Autodesk Inventor part; units mm, degrees
(part 3 of 3)
  line L283 (26.9505, 35.0379) -> (29.2108, 35.0457)
  line L284 (31.5582, 39.3166) -> (31.5476, 42.4293)
  line L285 (31.5596, 38.9092) -> (26.3728, 35.924)
  line L286 (26.3714, 36.3314) -> (31.5582, 39.3166)
  line L287 (31.5476, 42.4293) -> (21.5221, 36.4783)
  line L288 (31.7603, 43.0725) -> (21.0767, 36.7309)
  line L289 (19.9586, 37.4674) -> (31.7966, 44.45)
  line L290 (31.9286, 42.4307) -> (31.9366, 40.0825)
  line L291 (31.9286, 42.4307) -> (31.9285, 42.4639)
  line L292 (31.7966, 44.45) -> (43.6866, 37.5937)
  line L293 (42.5183, 36.9086) -> (31.7603, 43.0725)
  line L294 (42.0747, 36.6505) -> (31.9285, 42.4639)
  line L295 (31.5636, 37.7372) -> (31.5596, 38.9092)
  arc A47 (31.5636, 37.7372) -> (31.9446, 37.7385) centre (31.7568, 36.9673) ccw
  line L296 (38.1142, 35.719) -> (38.1116, 36.4859)
  arc A48 (38.7601, 35.0783) -> (38.1142, 35.719) centre (37.9285, 34.8858) ccw
  line L297 (37.7332, 36.2932) -> (37.7351, 35.7209)
  line L298 (38.3728, 25.9055) -> (37.1595, 25.9014)
  line L299 (37.1582, 26.2824) -> (38.3715, 26.2865)
  line L300 (37.1595, 25.9014) -> (37.1582, 26.2824)
  line L301 (36.3108, 29.8585) -> (35.1678, 29.8546)
  line L302 (34.347, 26.7047) -> (35.1786, 26.7075)
  line L303 (35.1678, 29.8546) -> (35.1786, 26.7075)
  line L304 (35.1786, 26.7075) -> (35.2746, 26.7079)
  line L305 (36.3215, 26.7115) -> (36.3108, 29.8585)
  line L306 (36.3215, 26.7115) -> (37.1567, 26.7143)
  line L307 (34.3505, 25.6887) -> (34.347, 26.7047)
  line L308 (37.1602, 25.6983) -> (34.3505, 25.6887)
  line L309 (37.1567, 26.7143) -> (37.1602, 25.6983)
  arc A49 (38.6709, 29.0181) -> (38.3681, 27.268) centre (38.5556, 28.1368) ccw
  line L310 (29.165, 23.8796) -> (25.8795, 23.8684)
  line L311 (23.0676, 23.4777) -> (29.1663, 23.4986)
  line L312 (30.8931, 30.8743) -> (32.1631, 30.8786)
  line L313 (33.9093, 28.7073) -> (32.6624, 28.703)
  line L314 (32.6638, 28.2849) -> (32.6624, 28.703)
  line L315 (33.9107, 28.2892) -> (32.6638, 28.2849)
  line L316 (33.9142, 27.2732) -> (33.9107, 28.2892)
  line L317 (32.6585, 29.846) -> (31.5155, 29.8421)
  line L318 (31.5155, 29.8421) -> (33.9054, 29.8503)
  line L319 (31.5194, 28.6991) -> (31.5155, 29.8421)
  line L320 (32.6673, 27.2689) -> (33.9142, 27.2732)
  line L321 (32.6688, 26.818) -> (32.6673, 27.2689)
  line L322 (33.9158, 26.8222) -> (32.6688, 26.818)
  line L323 (31.5155, 29.8421) -> (31.5298, 25.6711)
  line L324 (33.9197, 25.6792) -> (33.9158, 26.8222)
  line L325 (31.5298, 25.6711) -> (33.9197, 25.6792)
  line L326 (31.5298, 25.6711) -> (32.6728, 25.675)
  line L327 (31.5258, 26.8141) -> (31.5298, 25.6711)
  line L328 (31.5208, 28.281) -> (31.5243, 27.265)
  line L329 (39.2326, 22.7164) -> (42.1166, 24.4043)
  line L330 (38.7647, 22.7148) -> (39.2326, 22.7164)
  line L331 (35.6693, 22.7042) -> (38.3837, 22.7135)
  line L332 (35.2848, 23.7486) -> (35.2883, 22.7029)
  circle A50 centre (35.4727, 24.4871) radius 0.3175
  arc A51 (35.6658, 23.7499) -> (35.2848, 23.7486) centre (35.4727, 24.4871) ccw
  line L333 (32.0618, 22.6919) -> (35.2883, 22.7029)
  line L334 (35.6693, 22.7042) -> (35.6658, 23.7499)
  line L335 (38.5779, 22.3332) -> (32.0667, 22.3109)
  line L336 (32.0667, 22.3109) -> (38.5779, 22.3332)
  line L337 (31.8964, 17.907) -> (42.562, 24.1393)
  line L338 (43.6957, 23.5059) -> (31.8713, 16.6404)
  line L339 (32.0796, 18.5298) -> (38.5779, 22.3332)
  line L340 (32.0761, 18.5277) -> (38.5779, 22.3332)
  line L341 (32.0667, 22.3109) -> (32.0796, 18.5298)
  line L342 (31.75, 80.4139) -> (44.6823, 72.8573)
  line L343 (44.6823, 72.8573) -> (54.0323, 76.3351)
  line L344 (54.0323, 76.3351) -> (63.5, 70.8029)
  line L345 (31.75, 72.2052) -> (31.75, 88.9) construction
  line L346 (31.75, 80.4139) -> (18.8177, 72.8573)
  line L347 (18.8177, 72.8573) -> (9.4677, 76.3351)
  line L348 (9.4677, 76.3351) -> (0, 70.8029)
  line L349 (29.1432, 44.45) -> (63.5, 44.45) construction
  line L350 (9.4677, 12.5649) -> (0, 18.0971)
  line L351 (18.8177, 16.0427) -> (9.4677, 12.5649)
  line L352 (31.75, 8.4861) -> (18.8177, 16.0427)
  line L353 (31.75, 8.4861) -> (44.6823, 16.0427)
  line L354 (44.6823, 16.0427) -> (54.0323, 12.5649)
  line L355 (54.0323, 12.5649) -> (63.5, 18.0971)
  line L356 (0, 51.1737) -> (17.8526, 51.1737)
  line L357 (17.8526, 51.1737) -> (29.1432, 44.45)
  line L358 (17.8526, 37.7263) -> (29.1432, 44.45)
  line L359 (0, 37.7263) -> (17.8526, 37.7263)
  line L360 (63.5, 51.1737) -> (45.6474, 51.1737)
  line L361 (45.6474, 51.1737) -> (34.3568, 44.45)
  line L362 (45.6474, 37.7263) -> (34.3568, 44.45)
  line L363 (63.5, 37.7263) -> (45.6474, 37.7263)
  point P0 (0, 0)
  point P1 (31.7785, 58.3278)
  point P2 (31.8262, 30.4638)
  point P3 (-150.7587, 38.3711)
  point P4 (-161.1855, 44.542)
  point P5 (-156.3366, 47.458)
  point P6 (-155.762, 47.458)
  point P7 (-155.762, 49.0926)
  point P8 (-150.6894, 62.2724)
  point P9 (-155.762, 49.4736)
  point P10 (-154.619, 45.7468)
  point P11 (-155.762, 46.7628)
  point P12 (-155.762, 47.077)
  point P13 (-145.5843, 54.5372)
  point P14 (-145.5843, 54.9182)
  point P15 (-155.762, 53.9477)
  point P16 (-155.762, 53.5667)
  point P17 (-150.0718, 50.9582)
  point P18 (-151.2148, 52.1012)
  point P19 (-151.2148, 52.5193)
  point P20 (-150.7519, 34.4405)
  point P21 (-161.1576, 28.2339)
  point P22 (-155.7186, 23.702)
  point P23 (-155.7242, 25.3366)
  point P24 (-156.2988, 25.3346)
  point P25 (-155.7033, 19.2279)
  point P26 (-155.702, 18.8469)
  point P27 (-145.521, 17.9112)
  point P28 (-145.5223, 18.2922)
  point P29 (-155.7255, 25.7176)
  point P30 (-155.7266, 26.0318)
  point P31 (-154.587, 27.0517)
  point P32 (-155.7173, 23.321)
  point P33 (-151.1611, 20.7089)
  point P34 (-150.022, 21.8558)
  point P35 (-119.1805, 10.1069)
  point P36 (-182.6805, 10.1069)
  point P37 (-182.6805, 62.8127)
  dimension "d27" = 63.5
  dimension "d28" = 88.9
  constraints: 728 end point, 89 parallel, 64 point on circle, 50 centre point, 37 horizontal, 22 point on line, 21 perpendicular, 20 coincident, 17 symmetric about line, 5 vertical, 4 collinear, 2 midpoint, 11 other
  measures "d27" distance of L2.end L1.end
  measures "d28" distance of L1.end L0.end
extrude "Extrusion5" add sketch "Sketch6" against normal blind 0.8 separate body contours L109 L133 L129 L127 L155 L144 | L288 L293 L207 L337 L189 L182
sketch "Sketch7" plane through (0, 0, 0.4) normal (0, 0, 1) x (1, 0, 0)
  line L0 (63.5, 0) -> (63.5, 18.0971) projected
  line L1 (63.5, 0) -> (0, 0)
  line L2 (0, 0) -> (0, 88.9)
  line L3 (0, 88.9) -> (63.5, 88.9)
  line L4 (63.5, 88.9) -> (63.5, 0)
  constraints: 8 end point, 2 parallel, 1 horizontal, 1 perpendicular
extrude "Extrusion6" add sketch "Sketch7" along normal blind 0.4 bodies 2
sketch "Sketch8" plane through (0, 0, 0.8) normal (0, 0, 1) x (1, 0, 0)
  line L0 (5.5444, 85.725) -> (13.9597, 85.725) construction
  line L1 (13.9597, 85.725) -> (13.9597, 77.1126) construction
  line L2 (13.9597, 77.1126) -> (5.5444, 77.1126) construction
  line L3 (5.5444, 77.1126) -> (5.5444, 85.725) construction
  line L4 (49.5403, 22.4335) -> (53.7479, 24.8628)
  line L5 (53.7479, 24.8628) -> (57.9556, 22.4335)
  line L6 (57.9556, 22.4335) -> (57.9556, 17.5749)
  line L7 (57.9556, 17.5749) -> (53.7479, 15.1456)
  line L8 (53.7479, 15.1456) -> (49.5403, 17.5749)
  line L9 (49.5403, 17.5749) -> (49.5403, 22.4335)
  line L10 (63.5, 88.9) -> (0, 88.9) construction
  line L11 (63.5, 51.1737) -> (63.5, 37.7263) construction
  line L12 (63.5, 44.45) -> (0, 44.45) construction
  line L13 (0, 37.7263) -> (0, 51.1737) construction
  line L14 (0, 0) -> (63.5, 0) construction
  line L15 (31.75, 0) -> (31.75, 88.9) construction
  line L16 (13.9597, 71.3251) -> (13.9597, 66.4665)
  line L17 (5.5444, 66.4665) -> (5.5444, 71.3251)
  line L18 (13.9597, 66.4665) -> (9.7521, 64.0372)
  line L19 (9.7521, 64.0372) -> (5.5444, 66.4665)
  line L20 (5.5444, 71.3251) -> (9.7521, 73.7544)
  line L21 (9.7521, 73.7544) -> (13.9597, 71.3251)
  line L22 (57.9556, 3.175) -> (49.5403, 3.175) construction
  line L23 (49.5403, 3.175) -> (49.5403, 13.0967) construction
  line L24 (49.5403, 13.0967) -> (57.9556, 13.0967) construction
  line L25 (57.9556, 13.0967) -> (57.9556, 3.175) construction
  line L26 (23.2632, 24.9041) -> (31.75, 29.804)
  line L27 (31.75, 29.804) -> (40.2368, 24.9041)
  line L28 (40.2368, 24.9041) -> (40.2368, 15.1043)
  line L29 (40.2368, 15.1043) -> (31.75, 10.2044)
  line L30 (31.75, 10.2044) -> (23.2632, 15.1043)
  line L31 (23.2632, 15.1043) -> (23.2632, 24.9041)
  line L32 (40.2368, 73.7957) -> (31.75, 78.6956)
  line L33 (31.75, 78.6956) -> (23.2632, 73.7957)
  line L34 (23.2632, 63.9959) -> (31.75, 59.096)
  line L35 (23.2632, 73.7957) -> (23.2632, 63.9959)
  line L36 (31.75, 59.096) -> (40.2368, 63.9959)
  line L37 (40.2368, 63.9959) -> (40.2368, 73.7957)
  line L38 (12.9466, 76.2318) -> (6.681, 76.2318)
  line L39 (6.681, 76.2318) -> (6.681, 77.6726)
  spline S0 degree 2 poles (6.681, 77.6726) (7.3561, 78.3066) (8.5582, 79.484) (9.1346, 80.1179) knots 0 0 0 1 2 2 2
  spline S1 degree 2 poles (9.1346, 80.1179) (10.2955, 81.3941) (11.1435, 82.9255) (11.1435, 83.7406) knots 0 0 0 1 2 2 2
  spline S2 degree 2 poles (11.1435, 83.7406) (11.1435, 84.1688) (10.88, 84.811) (10.6413, 85.0168) knots 0 0 0 1 2 2 2
  spline S3 degree 2 poles (10.6413, 85.0168) (10.4025, 85.2226) (9.7768, 85.4285) (9.398, 85.4285) knots 0 0 0 1 2 2 2
  spline S4 degree 2 poles (9.398, 85.4285) (9.0358, 85.4285) (8.2948, 85.2473) (7.9572, 85.1074) knots 0 0 0 1 2 2 2
  spline S5 degree 2 poles (7.9572, 85.1074) (7.669, 84.9921) (7.1338, 84.6628) (6.9692, 84.5475) knots 0 0 0 1 2 2 2
  line L40 (6.9692, 84.5475) -> (6.8951, 84.5475)
  line L41 (6.8951, 84.5475) -> (6.8951, 85.9966)
  spline S6 degree 2 poles (6.8951, 85.9966) (7.315, 86.2024) (8.8217, 86.6059) (9.4968, 86.6059) knots 0 0 0 1 2 2 2
  spline S7 degree 2 poles (9.4968, 86.6059) (10.9212, 86.6059) (12.5267, 85.0991) (12.5267, 83.8147) knots 0 0 0 1 2 2 2
  spline S8 degree 2 poles (12.5267, 83.8147) (12.5267, 83.2137) (12.2468, 82.2092) (11.9998, 81.7811) knots 0 0 0 1 2 2 2
  spline S9 degree 2 poles (11.9998, 81.7811) (11.7528, 81.3365) (11.0365, 80.4637) (10.6413, 80.0438) knots 0 0 0 1 2 2 2
  spline S10 degree 2 poles (10.6413, 80.0438) (9.9991, 79.344) (8.4265, 77.8455) (7.9572, 77.4092) knots 0 0 0 1 2 2 2
  line L42 (7.9572, 77.4092) -> (12.9466, 77.4092)
  line L43 (12.9466, 77.4092) -> (12.9466, 76.2318)
  line L44 (50.5534, 13.3229) -> (56.819, 13.3229)
  line L45 (56.819, 13.3229) -> (56.819, 11.882)
  spline S11 degree 2 poles (56.819, 11.882) (56.1439, 11.2481) (54.9418, 10.0707) (54.3654, 9.4367) knots 0 0 0 1 2 2 2
  spline S12 degree 2 poles (54.3654, 9.4367) (53.2045, 8.1605) (52.3565, 6.6291) (52.3565, 5.814) knots 0 0 0 1 2 2 2
  spline S13 degree 2 poles (52.3565, 5.814) (52.3565, 5.3859) (52.62, 4.7437) (52.8587, 4.5378) knots 0 0 0 1 2 2 2
  spline S14 degree 2 poles (52.8587, 4.5378) (53.0975, 4.332) (53.7232, 4.1262) (54.102, 4.1262) knots 0 0 0 1 2 2 2
  spline S15 degree 2 poles (54.102, 4.1262) (54.4642, 4.1262) (55.2052, 4.3073) (55.5428, 4.4473) knots 0 0 0 1 2 2 2
  spline S16 degree 2 poles (55.5428, 4.4473) (55.831, 4.5625) (56.3662, 4.8919) (56.5308, 5.0072) knots 0 0 0 1 2 2 2
  line L46 (56.5308, 5.0072) -> (56.6049, 5.0072)
  line L47 (56.6049, 5.0072) -> (56.6049, 3.5581)
  spline S17 degree 2 poles (56.6049, 3.5581) (56.185, 3.3522) (54.6783, 2.9488) (54.0032, 2.9488) knots 0 0 0 1 2 2 2
  spline S18 degree 2 poles (54.0032, 2.9488) (52.5788, 2.9488) (50.9733, 4.4555) (50.9733, 5.7399) knots 0 0 0 1 2 2 2
  spline S19 degree 2 poles (50.9733, 5.7399) (50.9733, 6.341) (51.2532, 7.3454) (51.5002, 7.7736) knots 0 0 0 1 2 2 2
  spline S20 degree 2 poles (51.5002, 7.7736) (51.7472, 8.2182) (52.4635, 9.0909) (52.8587, 9.5108) knots 0 0 0 1 2 2 2
  spline S21 degree 2 poles (52.8587, 9.5108) (53.5009, 10.2107) (55.0735, 11.7091) (55.5428, 12.1455) knots 0 0 0 1 2 2 2
  line L48 (55.5428, 12.1455) -> (50.5534, 12.1455)
  line L49 (50.5534, 12.1455) -> (50.5534, 13.3229)
  point P0 (53.7479, 20.0042)
  point P1 (9.7521, 68.8958)
  point P2 (49.5403, 8.1358)
  point P3 (31.75, 20.0042)
  point P4 (31.75, 68.8958)
  dimension "d33" = 8.4153
  dimension "d34" = 8.4153
  dimension "d35" = 8.4153
  dimension "d41" = 3.175
  dimension "d42" = 3.175
  constraints: 52 end point, 7 symmetric about line, 5 midpoint, 4 vertical, 3 collinear, 1 point on line, 30 other
  measures "d33" distance between parallel lines of L3 L1
  measures "d34" distance between parallel lines of L17 L16
  measures "d35" distance from line of point (49.54, 8.136) L25
  measures "d41" distance between parallel lines of L10 L0
  measures "d42" distance between parallel lines of L14 L22
extrude "Extrusion7" cut sketch "Sketch8" against normal blind 0.4 bodies 2
sketch "Sketch9" plane through (0, 0, 0.4) normal (0, 0, 1) x (1, 0, 0)
  line L0 (12.9466, 77.4092) -> (12.9466, 76.2318) projected
  line L1 (12.9466, 76.2318) -> (6.681, 76.2318) projected
  line L2 (6.681, 76.2318) -> (6.681, 77.6726) projected
  spline S0 degree 2 poles (6.681, 77.6726) (7.3561, 78.3066) (8.5582, 79.484) (9.1346, 80.1179) knots 0 0 0 0.5 1 1 1 projected
  spline S1 degree 2 poles (9.1346, 80.1179) (10.2955, 81.3941) (11.1435, 82.9255) (11.1435, 83.7406) knots 0 0 0 0.5 1 1 1 projected
  spline S2 degree 2 poles (11.1435, 83.7406) (11.1435, 84.1688) (10.88, 84.811) (10.6413, 85.0168) knots 0 0 0 0.5 1 1 1 projected
  spline S3 degree 2 poles (10.6413, 85.0168) (10.4025, 85.2226) (9.7768, 85.4285) (9.398, 85.4285) knots 0 0 0 0.5 1 1 1 projected
  spline S4 degree 2 poles (9.398, 85.4285) (9.0358, 85.4285) (8.2948, 85.2473) (7.9572, 85.1074) knots 0 0 0 0.5 1 1 1 projected
  spline S5 degree 2 poles (7.9572, 85.1074) (7.669, 84.9921) (7.1338, 84.6628) (6.9692, 84.5475) knots 0 0 0 0.5 1 1 1 projected
  line L3 (6.9692, 84.5475) -> (6.8951, 84.5475) projected
  line L4 (6.8951, 84.5475) -> (6.8951, 85.9966) projected
  spline S6 degree 2 poles (6.8951, 85.9966) (7.315, 86.2024) (8.8217, 86.6059) (9.4968, 86.6059) knots 0 0 0 0.5 1 1 1 projected
  spline S7 degree 2 poles (9.4968, 86.6059) (10.9212, 86.6059) (12.5267, 85.0991) (12.5267, 83.8147) knots 0 0 0 0.5 1 1 1 projected
  spline S8 degree 2 poles (12.5267, 83.8147) (12.5267, 83.2137) (12.2468, 82.2092) (11.9998, 81.7811) knots 0 0 0 0.5 1 1 1 projected
  spline S9 degree 2 poles (11.9998, 81.7811) (11.7528, 81.3365) (11.0365, 80.4637) (10.6413, 80.0438) knots 0 0 0 0.5 1 1 1 projected
  spline S10 degree 2 poles (10.6413, 80.0438) (9.9991, 79.344) (8.4265, 77.8455) (7.9572, 77.4092) knots 0 0 0 0.5 1 1 1 projected
  line L5 (7.9572, 77.4092) -> (12.9466, 77.4092) projected
  line L6 (23.2632, 24.9041) -> (31.75, 29.804) projected
  line L7 (31.75, 29.804) -> (40.2368, 24.9041) projected
  line L8 (40.2368, 24.9041) -> (40.2368, 15.1043) projected
  line L9 (40.2368, 15.1043) -> (31.75, 10.2044) projected
  line L10 (31.75, 10.2044) -> (23.2632, 15.1043) projected
  line L11 (23.2632, 15.1043) -> (23.2632, 24.9041) projected
  line L12 (9.7521, 73.7544) -> (13.9597, 71.3251) projected
  line L13 (13.9597, 71.3251) -> (13.9597, 66.4665) projected
  line L14 (13.9597, 66.4665) -> (9.7521, 64.0372) projected
  line L15 (9.7521, 64.0372) -> (5.5444, 66.4665) projected
  line L16 (5.5444, 66.4665) -> (5.5444, 71.3251) projected
  line L17 (5.5444, 71.3251) -> (9.7521, 73.7544) projected
  line L18 (57.9556, 17.5749) -> (53.7479, 15.1456) projected
  line L19 (53.7479, 15.1456) -> (49.5403, 17.5749) projected
  line L20 (49.5403, 17.5749) -> (49.5403, 22.4335) projected
  line L21 (49.5403, 22.4335) -> (53.7479, 24.8628) projected
  line L22 (53.7479, 24.8628) -> (57.9556, 22.4335) projected
  line L23 (57.9556, 22.4335) -> (57.9556, 17.5749) projected
  line L24 (31.75, 78.6956) -> (40.2368, 73.7957) projected
  line L25 (40.2368, 73.7957) -> (40.2368, 63.9959) projected
  line L26 (40.2368, 63.9959) -> (31.75, 59.096) projected
  line L27 (31.75, 59.096) -> (23.2632, 63.9959) projected
  line L28 (23.2632, 63.9959) -> (23.2632, 73.7957) projected
  line L29 (23.2632, 73.7957) -> (31.75, 78.6956) projected
  line L30 (50.5534, 12.1455) -> (50.5534, 13.3229) projected
  line L31 (50.5534, 13.3229) -> (56.819, 13.3229) projected
  line L32 (56.819, 13.3229) -> (56.819, 11.882) projected
  spline S11 degree 2 poles (56.819, 11.882) (56.1439, 11.2481) (54.9418, 10.0707) (54.3654, 9.4367) knots 0 0 0 0.5 1 1 1 projected
  spline S12 degree 2 poles (54.3654, 9.4367) (53.2045, 8.1605) (52.3565, 6.6291) (52.3565, 5.814) knots 0 0 0 0.5 1 1 1 projected
  spline S13 degree 2 poles (52.3565, 5.814) (52.3565, 5.3859) (52.62, 4.7437) (52.8587, 4.5378) knots 0 0 0 0.5 1 1 1 projected
  spline S14 degree 2 poles (52.8587, 4.5378) (53.0975, 4.332) (53.7232, 4.1262) (54.102, 4.1262) knots 0 0 0 0.5 1 1 1 projected
  spline S15 degree 2 poles (54.102, 4.1262) (54.4642, 4.1262) (55.2052, 4.3073) (55.5428, 4.4473) knots 0 0 0 0.5 1 1 1 projected
  spline S16 degree 2 poles (55.5428, 4.4473) (55.831, 4.5625) (56.3662, 4.8919) (56.5308, 5.0072) knots 0 0 0 0.5 1 1 1 projected
  line L33 (56.5308, 5.0072) -> (56.6049, 5.0072) projected
  line L34 (56.6049, 5.0072) -> (56.6049, 3.5581) projected
  spline S17 degree 2 poles (56.6049, 3.5581) (56.185, 3.3522) (54.6783, 2.9488) (54.0032, 2.9488) knots 0 0 0 0.5 1 1 1 projected
  spline S18 degree 2 poles (54.0032, 2.9488) (52.5788, 2.9488) (50.9733, 4.4555) (50.9733, 5.7399) knots 0 0 0 0.5 1 1 1 projected
  spline S19 degree 2 poles (50.9733, 5.7399) (50.9733, 6.341) (51.2532, 7.3454) (51.5002, 7.7736) knots 0 0 0 0.5 1 1 1 projected
  spline S20 degree 2 poles (51.5002, 7.7736) (51.7472, 8.2182) (52.4635, 9.0909) (52.8587, 9.5108) knots 0 0 0 0.5 1 1 1 projected
  spline S21 degree 2 poles (52.8587, 9.5108) (53.5009, 10.2107) (55.0735, 11.7091) (55.5428, 12.1455) knots 0 0 0 0.5 1 1 1 projected
  line L35 (55.5428, 12.1455) -> (50.5534, 12.1455) projected
  line L36 (0, 88.9) -> (0, 0) projected
  line L37 (0, 0) -> (63.5, 0) projected
  line L38 (63.5, 0) -> (63.5, 88.9) projected
  line L39 (63.5, 88.9) -> (0, 88.9) projected
  point P0 (40.2368, 67.2462)
  constraints: 22 other
extrude "Extrusion8" add sketch "Sketch9" along normal blind 0.4 contours L0 L1 L2 S0 S1 S2 S3 S4 S5 L3 L4 S6 S7 S8 S9 S10 L5 | L6 L7 L8 L9 L10 L11 | L12 L13 L14 L15 L16 L17 | L18 L19 L20 L21 L22 L23 | L24 L25 L26 L27 L28 L29 | L30 L31 L32 S11 S12 S13 S14 S15 S16 L33 L34 S17 S18 S19 S20 S21 L35 bodies 1
fillet "Fillet1" radius 3.175 8 edges at (0, 0, 0.2) (63.5, 0, 0.2) (63.5, 88.9, 0.2) (0, 88.9, 0.2) (0, 0, 0.6) (63.5, 0, 0.6) (63.5, 88.9, 0.6) (0, 88.9, 0.6)
body "Solid1"
body "Solid2"
body "Solid3"
body "Solid4"
